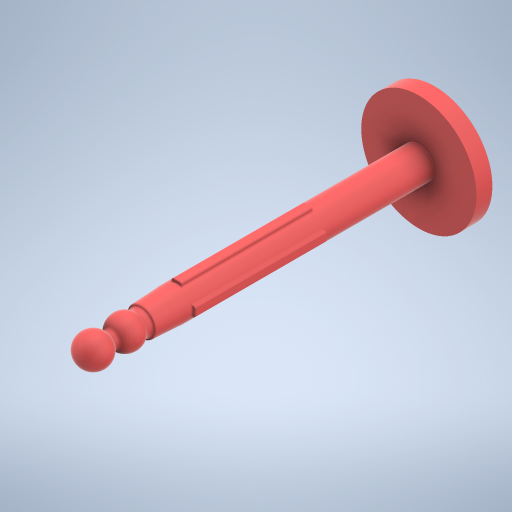
# Autodesk Inventor part: Pieza1
Saved by Autodesk Inventor 2024 (Build 280153000, 153)
## iProperties
Created: 2023-07-06
Part Number: Pieza1
Material: Plástico ABS
Document SubType Name: Modeling
Designer: Arthur
Density: 1.06 g/cm^3
Appearance: Suave - Rojo
Author: Arthur
Autodesk Inventor part; units mm, degrees
ref_plane "YZ Plane" through (0, 0, 0) normal (1, 0, 0) x (0, 1, 0)
ref_plane "XZ Plane" through (0, 0, 0) normal (0, 1, 0) x (-1, 0, 0)
sketch "Boceto1" plane through (0, 0, 0) normal (0, 0, 1) x (1, 0, 0)
  circle A0 centre (0, 0) radius 7.25
  dimension "d0" = 14.5
  constraints: 1 centre point, 1 coincident
  measures "d0" diameter of A0
extrude "Extrusión1" add sketch "Boceto1" along normal blind 2
sketch "Boceto2" plane through (0, 0, 2) normal (0, 0, 1) x (1, 0, 0)
  circle A0 centre (0, 0) radius 2
  dimension "d3" = 4
  constraints: 1 centre point, 1 coincident
  measures "d3" diameter of A0
extrude "Extrusión2" add sketch "Boceto2" along normal blind 43
sketch "Boceto3" plane through (0, 0, 0) normal (1, 0, 0) x (0, 1, 0)
  line L0 (2, 45) -> (-2, 45) projected
  line L1 (-2, 2) -> (2, 2) projected
  line L2 (-2, 2) -> (-2, 45) projected
  line L3 (2, 45) -> (-2, 45)
  line L4 (-2, 45) -> (-2, 41)
  line L5 (2, 41) -> (2, 45)
  arc A0 (1.2, 41.4) -> (-1.2, 41.4) centre (0, 43) ccw
  line L6 (-2, 41) -> (-2, 37)
  line L7 (-1.8, 37) -> (1.8, 37)
  line L8 (2, 37) -> (2, 41)
  arc A1 (-1.2, 40.6) -> (1.2, 40.6) centre (0, 39) ccw
  line L9 (0, 45) -> (0, 0)
  arc A2 (1.2, 41.4) -> (1.2, 40.6) centre (1.5, 41) ccw
  arc A3 (-1.2, 40.6) -> (-1.2, 41.4) centre (-1.5, 41) ccw
  line L10 (2, 45) -> (-2, 45)
  line L11 (-2, 45) -> (-2, 37)
  line L12 (-1.8, 37) -> (1.8, 37)
  line L13 (2, 37) -> (2, 45)
  line L14 (1.8, 37) -> (1, 37)
  line L15 (-1.8, 37) -> (-1, 37)
  line L16 (0, 37) -> (1.6, 37)
  line L17 (2, 37) -> (2, 33)
  line L18 (0, 37) -> (1.8, 37)
  line L19 (1.8, 37) -> (2, 33)
  line L20 (0, 37) -> (-1.8, 37)
  line L21 (-1.8, 37) -> (-2, 33)
  arc A4 (1.6, 37.8) -> (1.6, 37) centre (2.4, 37.4) ccw
  arc A5 (-1.6, 37) -> (-1.6, 37.8) centre (-2.4, 37.4) ccw
  point P0 (-1.6, 37.8)
  point P1 (-2, 39)
  point P2 (2, 39)
  point P3 (2, 43)
  point P4 (0, 45)
  point P5 (-2, 43)
  dimension "d12" = 1.6
  dimension "d13" = 4
  dimension "d14" = 1.8
  dimension "d15" = 1.8
  constraints: 38 end point, 14 point on circle, 6 centre point, 5 point on line, 4 parallel, 3 perpendicular, 3 symmetric about line, 3 tangent, 2 horizontal, 2 midpoint, 1 vertical, 1 other
  measures "d12" distance of L16.end L16.start
  measures "d13" distance of L13.start L17.end
  measures "d14" distance of L7.end L16.start
  measures "d15" distance of L7.start L16.start
revolve "Revolución1" cut sketch "Boceto3" angle 360 about axis through (0, 0, 45) along (0, 0, -1) contours L5 A0 L0 | A0 L2 L0 | L5 L8 A1 A2 A0 | A0 A3 A1 L2 | A5 L7 L21 L2 A1 | A1 L8 L17 L19 L7 A4
fillet "Empalme1" radius 0.2 1 edges at (0, 1.8, 37)
ref_plane "Plano de trabajo1" through (0, 0, 16) normal (0, 0, 1) x (1, 0, 0)
sketch "Boceto4" plane through (0, 0, 16) normal (0, 0, 1) x (1, 0, 0)
  circle A0 centre (0, 0) radius 2 projected
  line L0 (0.6, 1.9079) -> (0.6, 2.35)
  line L1 (0.6, 2.35) -> (-0.6, 2.35)
  line L2 (-0.6, 2.35) -> (-0.6, 1.9079)
  line L3 (0, 2) -> (0.6, 2.35) construction
  line L4 (0, 2) -> (-0.6, 2.35) construction
  arc A1 (0.6, 1.9079) -> (-0.6, 1.9079) centre (0, 0) ccw
  line L5 (-2.35, 0.6) -> (-2.35, -0.6)
  line L6 (-2.35, -0.6) -> (-1.9079, -0.6)
  arc A2 (-1.9079, 0.6) -> (-1.9079, -0.6) centre (0, 0) ccw
  line L7 (-1.9079, 0.6) -> (-2.35, 0.6)
  line L8 (-0.6, -2.35) -> (0.6, -2.35)
  line L9 (0.6, -2.35) -> (0.6, -1.9079)
  arc A3 (-0.6, -1.9079) -> (0.6, -1.9079) centre (0, 0) ccw
  line L10 (-0.6, -1.9079) -> (-0.6, -2.35)
  line L11 (2.35, -0.6) -> (2.35, 0.6)
  line L12 (2.35, 0.6) -> (1.9079, 0.6)
  arc A4 (1.9079, -0.6) -> (1.9079, 0.6) centre (0, 0) ccw
  line L13 (1.9079, -0.6) -> (2.35, -0.6)
  point P0 (-2, 0)
  point P1 (0, -2)
  point P2 (2, 0)
  dimension "d20" = 1.2
  dimension "d24" = 360
  constraints: 28 end point, 15 point on circle, 4 centre point, 1 coincident, 1 parallel, 41 other
  measures "d20" distance of L1.end L0.end
extrude "Extrusión3" add sketch "Boceto4" along normal blind 16.5 contours A0 L12 L11 L13 | A0 L2 L1 L0 | L9 L8 L10 A0 | A0 L6 L5 L7
fillet "Empalme2" radius 0.2 16 edges at (-0.6, 2.35, 24.25) (0.6, 2.35, 24.25) (-0.6, 1.9079, 24.25) (0.6, 1.9079, 24.25) (1.9079, 0.6, 24.25) (2.35, 0.6, 24.25) (2.35, -0.6, 24.25) (1.9079, -0.6, 24.25) (0.6, -2.35, 24.25) (0.6, -1.9079, 24.25) (-0.6, -1.9079, 24.25) (-0.6, -2.35, 24.25) (-2.35, 0.6, 24.25) (-2.35, -0.6, 24.25) (-1.9079, -0.6, 24.25) (-1.9079, 0.6, 24.25)
